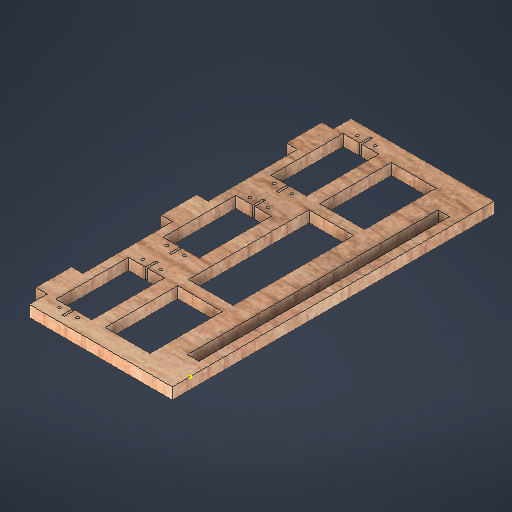
# Autodesk Inventor part: Servo Wall Skiba
Saved by Autodesk Inventor 2026.2 (Build 302298000, 298)
## iProperties
Created: 2025-11-09
Part Number: Servo Wall Skiba
Material: Generic
Document SubType Name: Modeling
Designer: Nick
Density: 1 g/cm^3
Appearance: Birch - Natural Polished
Author: Nick
Autodesk Inventor part; units mm, degrees
ref_plane "YZ Plane" through (0, 0, 0) normal (1, 0, 0) x (0, 1, 0)
ref_plane "XZ Plane" through (0, 0, 0) normal (0, 1, 0) x (-1, 0, 0)
ref_plane "XY Plane" through (0, 0, 0) normal (0, 0, 1) x (1, 0, 0)
sketch "Block1" plane through (0, 0, 0) normal (0, 0, 1) x (1, 0, 0)
  line L0 (-95.9812, 42.5391) -> (-55.4812, 42.5391)
  line L1 (-95.9812, 62.5391) -> (-95.9812, 42.5391)
  line L2 (-55.4812, 62.5391) -> (-95.9812, 62.5391)
  circle A0 centre (-65.4812, 52.5391) radius 2.75 construction
  arc A1 (-50.7312, 48.8391) -> (-50.7312, 46.2391) centre (-52.4812, 47.5391) ccw
  arc A2 (-50.7312, 58.8391) -> (-50.7312, 56.2391) centre (-52.4812, 57.5391) ccw
  arc A3 (-100.7311, 46.2391) -> (-100.7311, 48.8391) centre (-98.9812, 47.5391) ccw
  arc A4 (-100.7311, 56.2391) -> (-100.7311, 58.8391) centre (-98.9812, 57.5391) ccw
  circle A5 centre (-65.4812, 52.5391) radius 5 construction
  line L3 (-55.4812, 62.5391) -> (-55.4812, 42.5391)
  point P0 (-74.5923, 52.5391)
sketch "Sketch1" plane through (0, 0, 0) normal (0, 1, 0) x (-1, 0, 0)
  line L0 (75, 0) -> (55, 0)
  line L1 (55, 0) -> (55, -40.5)
  line L2 (55, -40.5) -> (75, -40.5)
  line L3 (75, -40.5) -> (75, 0)
  circle A0 centre (60, 3) radius 0.8
  circle A1 centre (70, 3) radius 0.8
  circle A2 centre (70, -43.5) radius 0.8
  circle A3 centre (60, -43.5) radius 0.8
  line L4 (55, 0) -> (64.4, 0)
  line L5 (64.4, 0) -> (65.6, 0)
  line L6 (65.6, 0) -> (65.6, 6)
  line L7 (65.6, 6) -> (64.4, 6)
  line L8 (64.4, 6) -> (64.4, 0)
  line L9 (75, -20.25) -> (55, -20.25) construction
  line L10 (64.4, -40.5) -> (65.6, -40.5)
  line L11 (65.6, -40.5) -> (65.6, -46.5)
  line L12 (65.6, -46.5) -> (64.4, -46.5)
  line L13 (64.4, -46.5) -> (64.4, -40.5)
  line L14 (0, 0) -> (55, 0) construction
  line L15 (0, -20) -> (0, 10) construction
  line L16 (0, 10) -> (80, 10)
  line L17 (80, 10) -> (80, -170)
  line L18 (80, -170) -> (0, -170)
  line L19 (0, -170) -> (0, 10)
  line L20 (75, -60) -> (55, -60)
  line L21 (65.6, -54) -> (64.4, -54)
  line L22 (65.6, -60) -> (65.6, -54)
  line L23 (64.4, -54) -> (64.4, -60)
  line L24 (55, -60) -> (64.4, -60)
  circle A4 centre (60, -57) radius 0.8
  circle A5 centre (70, -57) radius 0.8
  line L25 (75, -80.25) -> (55, -80.25) construction
  line L26 (64.4, -100.5) -> (65.6, -100.5)
  circle A6 centre (70, -103.5) radius 0.8
  line L27 (64.4, -106.5) -> (64.4, -100.5)
  line L28 (65.6, -106.5) -> (64.4, -106.5)
  line L29 (55, -100.5) -> (75, -100.5)
  circle A7 centre (60, -103.5) radius 0.8
  line L30 (75, -100.5) -> (75, -60)
  line L31 (55, -60) -> (55, -100.5)
  line L32 (65.6, -100.5) -> (65.6, -106.5)
  line L33 (64.4, -60) -> (65.6, -60)
  line L34 (75, -120) -> (55, -120)
  line L35 (65.6, -114) -> (64.4, -114)
  line L36 (65.6, -120) -> (65.6, -114)
  line L37 (64.4, -114) -> (64.4, -120)
  line L38 (55, -120) -> (64.4, -120)
  circle A8 centre (60, -117) radius 0.8
  circle A9 centre (70, -117) radius 0.8
  line L39 (75, -140.25) -> (55, -140.25) construction
  line L40 (64.4, -160.5) -> (65.6, -160.5)
  circle A10 centre (70, -163.5) radius 0.8
  line L41 (64.4, -166.5) -> (64.4, -160.5)
  line L42 (65.6, -166.5) -> (64.4, -166.5)
  line L43 (55, -160.5) -> (75, -160.5)
  circle A11 centre (60, -163.5) radius 0.8
  line L44 (75, -160.5) -> (75, -120)
  line L45 (55, -120) -> (55, -160.5)
  line L46 (65.6, -160.5) -> (65.6, -166.5)
  line L47 (64.4, -120) -> (65.6, -120)
  line L48 (0, 10) -> (5, 10)
  line L49 (5, 10) -> (5, -10)
  line L50 (5, -10) -> (0, -10)
  line L51 (0, -10) -> (0, 10)
  line L52 (5, -10) -> (11.35, -10)
  line L53 (11.35, -10) -> (11.35, -150)
  line L54 (11.35, -150) -> (5, -150)
  line L55 (5, -150) -> (5, -10)
  line L56 (80, 10) -> (47.5, 10)
  line L57 (47.5, 10) -> (47.5, 0)
  line L58 (47.5, 0) -> (80, 0)
  line L59 (80, 0) -> (80, 10)
  line L60 (47.5, 0) -> (22.5, 0)
  line L61 (22.5, 0) -> (22.5, -160)
  line L62 (22.5, -160) -> (47.5, -160)
  line L63 (47.5, -160) -> (47.5, 0)
  line L64 (47.5, -40.5) -> (22.5, -40.5)
  line L65 (22.5, -40.5) -> (22.5, -46.5)
  line L66 (22.5, -46.5) -> (47.5, -46.5)
  line L67 (47.5, -46.5) -> (47.5, -40.5)
  line L68 (47.5, -120) -> (22.5, -120)
  line L69 (22.5, -120) -> (22.5, -114)
  line L70 (22.5, -114) -> (47.5, -114)
  line L71 (47.5, -114) -> (47.5, -120)
  line L72 (75, -40.5) -> (75, 0)
  line L73 (55, -40.5) -> (75, -40.5)
  line L74 (55, 0) -> (55, -40.5)
  circle A12 centre (65, -10) radius 2.75 construction
  arc A13 (68.7, 4.75) -> (71.3, 4.75) centre (70, 3) ccw
  arc A14 (58.7, 4.75) -> (61.3, 4.75) centre (60, 3) ccw
  arc A15 (71.3, -45.25) -> (68.7, -45.25) centre (70, -43.5) ccw
  arc A16 (61.3, -45.25) -> (58.7, -45.25) centre (60, -43.5) ccw
  circle A17 centre (65, -10) radius 5 construction
  line L75 (55, 0) -> (75, 0)
  line L76 (75, -100.5) -> (75, -60)
  line L77 (55, -100.5) -> (75, -100.5)
  line L78 (55, -60) -> (55, -100.5)
  circle A18 centre (65, -70) radius 2.75 construction
  arc A19 (68.7, -55.25) -> (71.3, -55.25) centre (70, -57) ccw
  arc A20 (58.7, -55.25) -> (61.3, -55.25) centre (60, -57) ccw
  arc A21 (71.3, -105.25) -> (68.7, -105.25) centre (70, -103.5) ccw
  arc A22 (61.3, -105.25) -> (58.7, -105.25) centre (60, -103.5) ccw
  circle A23 centre (65, -70) radius 5 construction
  line L79 (55, -60) -> (75, -60)
  line L80 (75, -160.5) -> (75, -120)
  line L81 (55, -160.5) -> (75, -160.5)
  line L82 (55, -120) -> (55, -160.5)
  circle A24 centre (65, -130) radius 2.75 construction
  arc A25 (68.7, -115.25) -> (71.3, -115.25) centre (70, -117) ccw
  arc A26 (58.7, -115.25) -> (61.3, -115.25) centre (60, -117) ccw
  arc A27 (71.3, -165.25) -> (68.7, -165.25) centre (70, -163.5) ccw
  arc A28 (61.3, -165.25) -> (58.7, -165.25) centre (60, -163.5) ccw
  circle A29 centre (65, -130) radius 5 construction
  line L83 (55, -120) -> (75, -120)
  point P0 (55, -60)
  point P1 (64.4, -60)
  point P2 (65.6, 0)
  point P3 (65.6, -40.5)
  point P4 (64.4, -40.5)
  point P5 (64.4, 0)
  dimension "d40" = 40.5
  dimension "d41" = 20
  dimension "d42" = 3
  dimension "d43" = 3
  dimension "d44" = 5
  dimension "d45" = 10
  dimension "d46" = 10
  dimension "d60" = 60
  dimension "d38" = 0
  dimension "d47" = 1.6
  dimension "d48" = 1.6
  dimension "d49" = 1.6
  dimension "d50" = 9.4
  dimension "d51" = 1.2
  dimension "d52" = 6
  dimension "d54" = 0
  dimension "d55" = 30
  dimension "d56" = 80
  dimension "d57" = 180
  dimension "d65" = 0
  dimension "d66" = 10
  dimension "d74" = 5
  dimension "d75" = 5
  dimension "d76" = 6.35
  dimension "d77" = 140
  dimension "d88" = 32.5
  dimension "d89" = 25
  dimension "d90" = 160
  constraints: 144 end point, 18 parallel, 12 centre point, 10 horizontal, 9 perpendicular, 8 point on line, 4 symmetric about line, 4 vertical, 2 midpoint, 80 other
  measures "d47" diameter of A0
  measures "d48" diameter of A2
  measures "d49" diameter of A3
  measures "d50" distance of L0.end L4.end
  measures "d51" distance of L7.end L6.end
  measures "d52" distance of L6.end L5.end
  measures "d55" distance of L15.start L15.end
  measures "d56" distance of L17.end L18.end
  measures "d57" distance of L16.end L17.end
  measures "d65" horizontal distance of L14.start L15.end
  measures "d66" distance of L15.end L14.start
  measures "d74" distance between parallel lines of L17 L3
  measures "d75" distance of L49.end L50.end
  measures "d76" distance of L53.end L54.end
  measures "d77" distance of L52.end L53.end
  measures "d88" distance of L58.end L57.end
  measures "d89" distance of L62.end L61.end
  measures "d90" distance of L61.end L60.end
extrude "Extrusion1" add sketch "Sketch1" along normal blind 6.35 contours L63 L64 L61 L60 | L52 L53 L54 L55 | L58 L17 L18 L19 L50 L49 L16 L57 L1 L2 L13 L12 L11 L3 | L0 L6 L7 L8 L58 L57 L16 L17 | L49 L50 L19 L16 | L63 L66 L61 L64 | L63 L70 L61 L66 | L63 L68 L61 L70 | L63 L62 L61 L68
extrude "Extrusion3" cut sketch "Sketch1" along normal blind 6.35 contours L52 L53 L54 L55
sketch "Sketch3" plane through (0, 6.35, 0) normal (0, 1, 0) x (1, 0, 0)
  line L0 (0, 20) -> (6.35, 20) projected
  line L1 (0, 0) -> (6.35, 0)
  line L2 (6.35, 0) -> (6.35, 20)
  line L3 (6.35, 20) -> (0, 20)
  line L4 (0, 20) -> (0, 0)
  line L5 (0, 70) -> (6.35, 70) projected
  line L6 (0, 90) -> (6.35, 90) projected
  line L7 (0, 70) -> (6.35, 70)
  line L8 (6.35, 70) -> (6.35, 90)
  line L9 (6.35, 90) -> (0, 90)
  line L10 (0, 90) -> (0, 70)
  line L11 (0, 140) -> (6.35, 140) projected
  line L12 (0, 160) -> (6.35, 160) projected
  line L13 (0, 140) -> (6.35, 140)
  line L14 (6.35, 140) -> (6.35, 160)
  line L15 (6.35, 160) -> (0, 160)
  line L16 (0, 160) -> (0, 140)
  line L17 (-80, -10) -> (0, -10) construction
  line L18 (-40, -10) -> (-40, 201.7794) construction
  line L19 (-80, 20) -> (-86.35, 20)
  line L20 (-80, 0) -> (-86.35, 0)
  line L21 (-86.35, 0) -> (-86.35, 20)
  line L22 (-86.35, 20) -> (-80, 20)
  line L23 (-80, 20) -> (-80, 0)
  line L24 (-80, 70) -> (-86.35, 70)
  line L25 (-80, 90) -> (-86.35, 90)
  line L26 (-80, 70) -> (-86.35, 70)
  line L27 (-86.35, 70) -> (-86.35, 90)
  line L28 (-86.35, 90) -> (-80, 90)
  line L29 (-80, 90) -> (-80, 70)
  line L30 (-80, 140) -> (-86.35, 140)
  line L31 (-80, 160) -> (-86.35, 160)
  line L32 (-80, 140) -> (-86.35, 140)
  line L33 (-86.35, 140) -> (-86.35, 160)
  line L34 (-86.35, 160) -> (-80, 160)
  line L35 (-80, 160) -> (-80, 140)
  line L36 (-5, 150) -> (-5, 10) projected
  point P0 (3.175, 90)
  dimension "d82" = 6.35
  dimension "d83" = 10
  dimension "d84" = 50
  dimension "d85" = 5
  dimension "d86" = 50
  dimension "d87" = 6.35
  constraints: 60 end point, 17 symmetric about line, 6 parallel, 3 horizontal, 3 perpendicular, 2 midpoint, 1 vertical
  measures "d82" distance of L0.start L0.end
  measures "d83" distance of L17.end L1.start
  measures "d84" distance between parallel lines of L0 L5
  measures "d85" distance from line of L36 L0.start
  measures "d86" distance from line of point (3.175, 90) L11
  measures "d87" distance of L6.start L6.end
extrude "Extrusion4" add sketch "Sketch3" against normal blind 6.35 contours L23 L20 L21 L19 | L24 L27 L25 L29 | L30 L33 L31 L35
sketch "Sketch4" plane through (0, 6.35, 0) normal (0, 1, 0) x (1, 0, 0)
  point P0 (0, 0)
extrude "Extrusion5" cut sketch "Sketch1" along normal blind 6.35 contours L63 L64 L61 L60 | L63 L66 L61 L64 | L63 L70 L61 L66 | L63 L68 L61 L70 | L63 L62 L61 L68
extrude "Extrusion6" add sketch "Sketch1" along normal blind 6.35 contours L63 L66 L61 L64 | L63 L68 L61 L70
body "Solid1"
